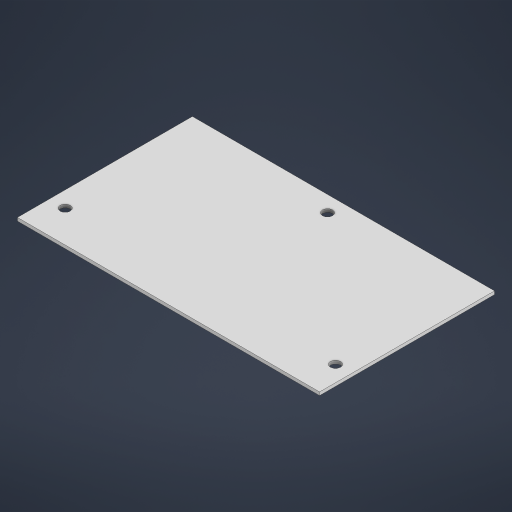
# Autodesk Inventor part: pcb
Saved by Autodesk Inventor 2024 (Build 280153000, 153)
## iProperties
Created: 2024-02-07
Part Number: pcb
Material: Všeobecné
Document SubType Name: Modeling
Designer: Simak
Density: 1 g/cm^3
Appearance: Výchozí
Author: Simak
Autodesk Inventor part; units mm, degrees
ref_plane "YZ Plane" through (0, 0, 0) normal (1, 0, 0) x (0, 1, 0)
ref_plane "XZ Plane" through (0, 0, 0) normal (0, 1, 0) x (-1, 0, 0)
ref_plane "XY Plane" through (0, 0, 0) normal (0, 0, 1) x (1, 0, 0)
sketch "Náčrt1" plane through (0, 0, 0) normal (0, 1, 0) x (-1, 0, 0)
  line L0 (-47.5, 27.5) -> (47.5, 27.5)
  line L1 (47.5, 27.5) -> (47.5, -27.5)
  line L2 (47.5, -27.5) -> (-47.5, -27.5)
  line L3 (-47.5, -27.5) -> (-47.5, 27.5)
  circle A0 centre (-42.5, 17.5) radius 1.6
  line L4 (-47.5, -27.5) -> (0, 0) construction
  line L5 (0, 0) -> (47.5, 27.5) construction
  line L6 (0, 0) -> (47.5, -27.5) construction
  circle A1 centre (42.5, 17.5) radius 1.6
  circle A2 centre (0, -22.5) radius 1.6
  dimension "d0" = 95
  dimension "d1" = 55
  dimension "d2" = 10
  dimension "d3" = 5
  dimension "d4" = 5
  dimension "d5" = 3.2
  dimension "d6" = 5
  constraints: 14 end point, 3 centre point, 2 equal length, 2 equal radius, 2 parallel, 1 horizontal, 1 horizontal alignment, 1 perpendicular, 1 vertical alignment
  measures "d0" distance of L0.start L0.end
  measures "d1" distance of L0.end L1.end
  measures "d2" distance from line of L0 A0.centre
  measures "d3" distance from line of L3 A0.centre
  measures "d4" distance from line of A1.centre L1
  measures "d5" diameter of A0
  measures "d6" distance from line of L2 A2.centre
extrude "Vysunutí1" add sketch "Náčrt1" along normal blind 1
equation "\"d4\" = d3"
equation "\"d6\" = d3"
